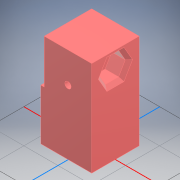
# Autodesk Inventor part: 000.001.001 - Уголок
Saved by Autodesk Inventor 2022 (Build 260153000, 153)
## iProperties
Created: 2022-02-23
Part Number: 000.001.001 - Уголок
Material: Пластик АБС
Document SubType Name: Modeling
Designer: Petrov Ivan
Density: 1.06 g/cm^3
Appearance: Гладкий — белый
Author: Petrov Ivan
Autodesk Inventor part; units mm, degrees
ref_plane "YZ Plane" through (0, 0, 0) normal (1, 0, 0) x (0, 1, 0)
ref_plane "XZ Plane" through (0, 0, 0) normal (0, 1, 0) x (-1, 0, 0)
ref_plane "XY Plane" through (0, 0, 0) normal (0, 0, 1) x (1, 0, 0)
sketch "Эскиз1" plane through (0, 0, 0) normal (0, 1, 0) x (-1, 0, 0)
  line L0 (-14, 14) -> (14, 14)
  line L1 (14, 14) -> (14, -14)
  line L2 (14, -14) -> (-14, -14)
  line L3 (-14, -14) -> (-14, 14)
  line L4 (-14, 14) -> (14, -14) construction
  line L5 (14, 14) -> (-14, -14) construction
  point P0 (0, 0)
  dimension "d0" = 28
  dimension "d1" = 28
  constraints: 12 end point, 2 midpoint, 2 parallel, 1 horizontal, 1 perpendicular
  measures "d0" distance of L1.end L2.end
  measures "d1" distance of L0.end L1.end
extrude "Выдавливание1" add sketch "Эскиз1" along normal blind 56
sketch "Эскиз2" plane through (0, 0, 0) normal (0, -1, 0) x (1, 0, 0)
  circle A0 centre (0, 0) radius 4
  constraints: 1 centre point, 1 coincident
extrude "Выдавливание2" cut sketch "Эскиз2" against normal blind 32
sketch "Эскиз3" plane through (-14, 0, -14) normal (-1, 0, 0) x (0, 0, 1)
  circle A0 centre (14, 46) radius 4 projected
  point P0 (14, 0)
extrude "Выдавливание3" cut sketch "Эскиз3" against normal through all
sketch "Эскиз4" plane through (14, 0, 14) normal (1, 0, 0) x (0, 0, -1)
  circle A0 centre (14, 46) radius 4 projected
  line L0 (6.2058, 46) -> (10.1029, 52.75)
  line L1 (10.1029, 52.75) -> (17.8971, 52.75)
  line L2 (17.8971, 52.75) -> (21.7942, 46)
  line L3 (21.7942, 46) -> (17.8971, 39.25)
  line L4 (17.8971, 39.25) -> (10.1029, 39.25)
  line L5 (10.1029, 39.25) -> (6.2058, 46)
  line L6 (0, 56) -> (28, 56) projected
  point P0 (14, 0)
  dimension "d8" = 13.5
  constraints: 12 end point, 1 coincident, 1 parallel, 13 other
  measures "d8" distance between parallel lines of L4 L1
extrude "Выдавливание4" cut sketch "Эскиз4" against normal blind 10
chamfer "Фаска1" distance 2 angle 45 6 edges at (14, 39.25, 0) (14, 42.625, -5.8457) (14, 49.375, -5.8457) (14, 52.75, 0) (14, 49.375, 5.8457) (14, 42.625, 5.8457)
ref_plane "РабПлоскость1" through (0, 22, 0) normal (0, -1, 0) x (1, 0, 0)
sketch "Эскиз5" plane through (0, 22, 0) normal (0, -1, 0) x (1, 0, 0)
  line L0 (0, 8.0829) -> (7, 4.0415)
  line L1 (7, 4.0415) -> (7, -4.0415)
  line L2 (7, -4.0415) -> (0, -8.0829)
  line L3 (0, -8.0829) -> (-7, -4.0415)
  line L4 (-7, -4.0415) -> (-7, 4.0415)
  line L5 (-7, 4.0415) -> (0, 8.0829)
  line L6 (0, 8.0829) -> (-14, 8.0829)
  line L7 (-14, -14) -> (-14, 14) projected
  line L8 (0, -8.0829) -> (-14, -8.0829)
  line L9 (-14, 8.0829) -> (-14, -8.0829)
  point P0 (0, 0)
  point P1 (0, 0)
  dimension "d15" = 14
  constraints: 18 end point, 2 point on line, 1 coincident, 1 collinear, 1 horizontal, 1 parallel, 13 other
  measures "d15" distance between parallel lines of L1 L4
extrude "Выдавливание5" cut sketch "Эскиз5" along normal mid plane 10
chamfer "Фаска2" distance 2 angle 45 4 edges at (-14, 27, 0) (-14, 22, 8.0829) (-14, 17, 0) (-14, 22, -8.0829)
sketch "Эскиз6" plane through (-14, 0, -14) normal (-1, 0, 0) x (0, 0, 1)
  line L0 (28, 0) -> (28, 56) projected
  line L1 (0, 0) -> (0, 56) projected
  line L2 (28, 0) -> (0, 0)
  line L3 (0, 0) -> (0, 30)
  line L4 (0, 30) -> (28, 30)
  line L5 (28, 30) -> (28, 0)
  line L6 (24.0829, 15) -> (24.0829, 29) projected
  line L7 (3.9171, 15) -> (24.0829, 15) projected
  line L8 (3.9171, 29) -> (3.9171, 15) projected
  line L9 (24.0829, 29) -> (3.9171, 29) projected
  point P0 (14, 0)
  point P1 (28, 30)
  dimension "d21" = 30
  constraints: 8 end point, 2 parallel, 1 horizontal, 1 perpendicular, 1 point on line
  measures "d21" distance of L2.end L3.end
extrude "Выдавливание6" add sketch "Эскиз6" along normal blind 2
sketch "Эскиз7" plane through (-14, 56, 14) normal (0, 0, 1) x (1, 0, 0)
  circle A0 centre (14, -18) radius 1.85 projected
  point P0 (14, -56)
extrude "Выдавливание7" cut sketch "Эскиз7" against normal blind 12
mirror "Зеркальное отражение1" about plane through (0, 0, 0) normal (0, 0, 1) of "Выдавливание7"
equation "\"d1\" = d0"
equation "\"d2\" = 2 * d0"
